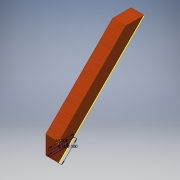
# Autodesk Inventor part: Angled Support
Saved by Autodesk Inventor 2016 (Build 200138000, 138)
## iProperties
Created: 2014-08-03
Part Number: Angled Support
Material: Generic
Document SubType Name: Modeling
Designer: Haden
Density: 1 g/cm^3
Appearance: Cherry - Natural Low Gloss
Author: Haden
Autodesk Inventor part; units mm, degrees
ref_plane "YZ Plane" through (0, 0, 0) normal (1, 0, 0) x (0, 1, 0)
ref_plane "XZ Plane" through (0, 0, 0) normal (0, 1, 0) x (-1, 0, 0)
ref_plane "XY Plane" through (0, 0, 0) normal (0, 0, 1) x (1, 0, 0)
sketch "Sketch1" plane through (0, 0, 0) normal (1, 0, 0) x (0, 1, 0)
  line L0 (0, 0) -> (-197.5656, 0)
  line L1 (-197.5656, 0) -> (716.8344, -914.4)
  line L2 (716.8344, -914.4) -> (716.8344, -716.8344)
  line L3 (716.8344, -716.8344) -> (0, 0)
  dimension "d1" = 139.7
  dimension "d2" = 914.4
  constraints: 8 end point, 2 perpendicular, 1 horizontal
  measures "d1" distance between parallel lines of L1 L3
  measures "d2" distance from line of L0.end L2
extrude "Extrusion1" add sketch "Sketch1" along normal blind 139.7
sketch "Sketch2" plane through (139.7, 0, 0) normal (1, 0, 0) x (0, 0, -1)
  line L0 (0, -197.5656) -> (914.4, 716.8344) projected
  line L1 (161.6446, -35.921) -> (-105.0554, -35.921)
  line L2 (110.8446, -86.721) -> (-105.0554, -86.721)
  point P0 (0, 0)
  dimension "d7" = 266.7
  dimension "d8" = 228.6
  dimension "d9" = 215.9
  constraints: 4 end point, 2 horizontal, 2 point on line, 1 vertical alignment
  measures "d7" distance of L1.start L1.end
  measures "d8" distance of L1.start L0.start
  measures "d9" distance of L2.start L2.end
body "Solid1"
